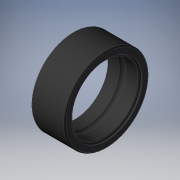
# Autodesk Inventor part: SKF_WBB1-8705-2RS1_or
Saved by Autodesk Inventor 2019 (Build 230136000, 136)
## iProperties
Created: 2023-07-31
Part Number: SKF_WBB1-8705-2RS1_or
Material: Generic
Catalog Web Link: www.cadenas.de
Description: BB1_001_101_or-Deep groove ball bearings
Vendor: SKF
Document SubType Name: Modeling
Designer: psAdmin
Manufacturer: SKF
Mass: 0.11751 g
Surface Area: 2.80901 cm^2
Volume: 0.11751 cm^3
Density: 1 g/cm^3
Appearance: PSOLRGB-175-175-175
Category: PARTsolutions
Company: SKF
Title: SKF_WBB1-8705-2RS1_or
Author: Cadenas PARTsolutions
Comments: Deep groove ball bearings
PSOL_IDENT_0: {$CADENAS_DATA/23d-libs/skf/bearings_units_and_housings/ball_bearings/deep_groove_ball_bearings/part
PSOL_IDENT_1: s/bb1_001_101_or.prj},193 {VTYP=3D},{NB=SKF_WBB1-8705-2RS1_or},{LINA=SKF_WBB1-8705-2RS1_or},{NN=BB1_
PSOL_IDENT_2: 001_101_or},{DATE=25.11.2022 05:56:16},{GEOMDATE=21.11.2022 10:24:00},{VERSION=},{LINEID=21140},{WBV
PSOL_IDENT_3: AR=},{WBNUMERIC=}  {NB=SKF_WBB1-8705-2RS1_or},{LINA=SKF_WBB1-8705-2RS1_or},{KT=DUMMY},{DESIGNATION=W
PSOL_IDENT_4: BB1-8705-2RS1},{R12=0.15},{DD=5.000},{D=10.000},{B=4.000},{C=},{CX=},{CXX=},{CA=0.000},{XXVARIANT=},
PSOL_IDENT_5: {XXDESIGN=Single row stainless steel},{XXSEALING=Contact seal on both sides},{DESIGN=dgbb2rs},{DESIG
PSOL_IDENT_6: NIR=dgbb2rs},{VARIANT=},{DD1=6.00},{DD2=6},{DD2X=},{DD2A=6.00},{D1=7.80},{D1X=0.00},{D2=8.4},{D2A=8.
PSOL_IDENT_7: 40},{D3=},{D3X=},{D3A=0.000},{D4=},{HH=0.000},{BB=0.000},{BBX=},{BBA=0.000},{FF=},{R0MAX=0.000},{R0=
PSOL_IDENT_8: 0.000},{PITCH=6.90},{DW=1.200},{DDAMIN=5.900},{DDAMAX=5.900},{DDBMIN=0.000},{DDBMAX=0.000},{DBMIN=0.
PSOL_IDENT_9: 000},{DAMAX=8.800},{BBAMIN=0.000},{CAMAX=0.000},{RAMAX=0.150},{LOAD1=0.247},{LOAD2=0.085},{LOAD3=0.0
PSOL_IDENT_10: 04},{SPEED1=0},{SPEED2=38000},{KR=0.015},{F0=7.600},{Z=8},{II=1},{MASS=0.001},{BEARING=WBB1-8705-2RS
PSOL_IDENT_11: 1},{RING=},{HELP=1.100},{HELP2=0.800},{DD1ALG=3.000},{YALG=3.000},{PITCH1=6.900},{DW1=1.200},{YALG1=
PSOL_IDENT_12: 3.900},{HALG1=1.100},{SH=3.000},{CU=0.560},{HALG=0.5},{B1=0},{SHIELDHELP=2},{D4A=0.000},{FFA=0.000},
PSOL_IDENT_13: {RS1=},{HELP3=0},{SUPPRESS=0}
NB: SKF_WBB1-8705-2RS1_or
NN: BB1_001_101_or
NT: Deep groove ball bearings
NBSYN: SKF_$DESIGNATION._or
LINA: SKF_WBB1-8705-2RS1_or
CATALOG: SKF
DESIGNATION: WBB1-8705-2RS1
R12: 0.15
DD: 5
D: 10
B: 4
XXDESIGN: Single row stainless steel
XXSEALING: Contact seal on both sides
DD1: 6
DD2: 6
D1: 7.8
D1X: 0
D2: 8.4
HH: 0
BB: 0
R0MAX: 0
R0: 0
PITCH: 6.9
DW: 1.2
DDAMIN: 5.9
DDAMAX: 5.9
DDBMIN: 0
DDBMAX: 0
DBMIN: 0
DAMAX: 8.8
BBAMIN: 0
CAMAX: 0
RAMAX: 0.15
LOAD1: 0.247
LOAD2: 0.085
LOAD3: 0.004
SPEED1: 0
SPEED2: 38000
KR: 0.015
F0: 7.6
Z: 8
II: 1
MASS: 0.001
BEARING: WBB1-8705-2RS1
HELP3: 0
SUPPRESS: 0
SUPPLIER: SKF
ARTICLENO: SKF_WBB1-8705-2RS1_or
BOMINFO: SKF_WBB1-8705-2RS1_or
CREATOR: CADENAS GmbH
Autodesk Inventor part; units mm, degrees
sketch "Sketch_9" plane through (0, 0, 0) normal (0, 0, 1) x (1, 0, 0)
  line L0 (50, 0) -> (-50, 0)
  line L1 (0, 4.85) -> (0, 4.2)
  line L2 (0, 4.2) -> (0.075, 4.2)
  arc A0 (0.225, 4.05) -> (0.075, 4.2) centre (0.075, 4.05) ccw
  line L3 (0.225, 4.05) -> (0.225, 3.9)
  line L4 (0.225, 3.9) -> (1.6031, 3.9)
  arc A1 (2.3969, 3.9) -> (1.6031, 3.9) centre (2, 3.45) ccw
  line L5 (2.3969, 3.9) -> (3.775, 3.9)
  line L6 (3.775, 3.9) -> (3.775, 4.05)
  arc A2 (3.925, 4.2) -> (3.775, 4.05) centre (3.925, 4.05) ccw
  line L7 (3.925, 4.2) -> (4, 4.2)
  line L8 (4, 4.2) -> (4, 4.85)
  arc A3 (4, 4.85) -> (3.85, 5) centre (3.85, 4.85) ccw
  line L9 (3.85, 5) -> (0.15, 5)
  arc A4 (0.15, 5) -> (0, 4.85) centre (0.15, 4.85) ccw
  constraints: 20 end point, 10 point on circle, 5 centre point
revolve "Revolution1" add sketch "Sketch_9" angle 360 about axis through (50, 0, 0) along (1, 0, 0)
ref_plane "or_XY" through (0, 0, 0) normal (0, 0, 1) x (1, 0, 0)
ref_plane "or_YZ" through (0, 0, 0) normal (1, 0, 0) x (0, 1, 0)
ref_plane "or_ZX" through (0, 0, 0) normal (0, 1, 0) x (0, 0, 1)
body "Solid1"
